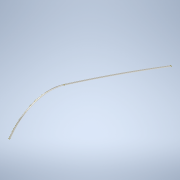
# Autodesk Inventor part: Wirebond
Saved by Autodesk Inventor 2022 (Build 260153000, 153)
## iProperties
Created: 2022-02-09
Part Number: Wirebond
Material: Generic
Document SubType Name: Modeling
Designer: Caleb
Density: 1 g/cm^3
Appearance: Silver
Author: Caleb
Autodesk Inventor part; units mm, degrees
ref_plane "YZ Plane" through (0, 0, 0) normal (1, 0, 0) x (0, 1, 0)
ref_plane "XZ Plane" through (0, 0, 0) normal (0, 1, 0) x (-1, 0, 0)
ref_plane "XY Plane" through (0, 0, 0) normal (0, 0, 1) x (1, 0, 0)
sketch "Sketch3" plane through (0, 0, 0) normal (0, 1, 0) x (-1, 0, 0)
  circle A0 centre (0, 0) radius 0.0125
  dimension "d10" = 0.025
  constraints: 1 centre point, 1 coincident
  measures "d10" diameter of A0
sketch "Sketch4" plane through (0, 0, 0) normal (1, 0, 0) x (0, 1, 0)
  line L0 (0, 0) -> (0, -0.15) construction
  line L1 (0, -0.15) -> (-0.33, -0.15) construction
  line L2 (-0.33, -0.15) -> (-0.33, -3) construction
  arc A0 (0.3608, -1.0118) -> (0, 0) centre (-0.4919, -0.7456) ccw
  arc A1 (-0.33, -3) -> (0.3608, -1.0118) centre (-31.1855, 8.8345) ccw
  dimension "d11" = 0.15
  dimension "d12" = 0.33
  dimension "d13" = 2.85
  dimension "d14" = 90
  constraints: 6 end point, 4 point on circle, 2 centre point, 2 perpendicular, 1 tangent, 1 vertical
  measures "d11" distance of L0.start L0.end
  measures "d12" distance of L0.end L1.end
  measures "d13" distance of L1.end L2.end
  measures "d14" angle of L2 L1
sweep "Sweep1" add profiles "Sketch3" path "Sketch4"
body "Solid1"
